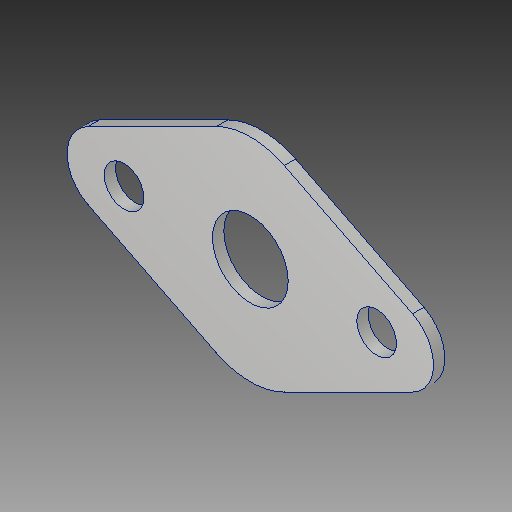
# Autodesk Inventor part: Maintient roulement
Saved by Autodesk Inventor 2017 (Build 210142000, 142)
## iProperties
Company: FABLAB Frenchmakers
Part Number: Maintient roulement
Material: Aluminium
Document SubType Name: Modeling
Designer: FABLAB Frenchmakers
Density: 2.7 g/cm^3
Appearance: Aluminium - Plat(2)
Mass: 0.653954 g
Surface Area: 6.35876 cm^2
Volume: 0.242205 cm^3
Stock Number: 1420-01-08
Project: 1420 Vauban 3D XL
Catalog Web Link: http://frenchmakers.com/
Autodesk Inventor part; units mm, degrees
ref_plane "YZ Plane" through (0, 0, 0) normal (1, 0, 0) x (0, 1, 0)
ref_plane "XZ Plane" through (0, 0, 0) normal (0, 1, 0) x (-1, 0, 0)
ref_plane "XY Plane" through (0, 0, 0) normal (0, 0, 1) x (1, 0, 0)
sketch "Esquisse1" plane through (0, 0, 0) normal (0, 0, 1) x (1, 0, 0)
  line L0 (-12.8425, 2.6828) -> (-2.685, 7.7657)
  line L1 (2.685, 7.7657) -> (12.8425, 2.6828)
  line L2 (12.8425, -2.6828) -> (2.685, -7.7657)
  line L3 (-2.685, -7.7657) -> (-12.8425, -2.6828)
  arc A0 (2.685, 7.7657) -> (-2.685, 7.7657) centre (0, 2.4) ccw
  arc A1 (-2.685, -7.7657) -> (2.685, -7.7657) centre (0, -2.4) ccw
  arc A2 (-12.8425, 2.6828) -> (-12.8425, -2.6828) centre (-11.5, 0) ccw
  arc A3 (12.8425, -2.6828) -> (12.8425, 2.6828) centre (11.5, 0) ccw
  point P0 (0, 0)
  point P1 (0, 9.1093)
  point P2 (18.2039, 0)
  point P3 (0, -9.1093)
  point P4 (-18.2039, 0)
  dimension "d0" = 6
  dimension "d1" = 3
  dimension "d2" = 29
  dimension "d3" = 16.8
  constraints: 8 end point, 8 point on circle, 8 point on line, 8 tangent, 4 centre point, 3 horizontal alignment, 2 equal length, 2 equal radius, 2 vertical alignment
  measures "d0" radius of A0
  measures "d1" radius of A2
extrude "Extrusion1" add sketch "Esquisse1" along normal blind 0.9
sketch "Esquisse2" plane through (0, 0, 0.9) normal (0, 0, 1) x (1, 0, 0)
  point P0 (0, 0)
  point P1 (0, 0)
  constraints: 1 coincident
hole "Perçage D6" at (0, 0, 0.9) direction (0, 0, -1) diameter 6 end through all
sketch "Esquisse3" plane through (0, 0, 0.9) normal (0, 0, 1) x (1, 0, 0)
  point P0 (0, 0)
  point P1 (-10, 0)
  point P2 (10, 0)
  dimension "d13" = 20
  dimension "d21" = 10
  constraints: 2 horizontal alignment
  measures "d13" distance of point (10, 0) point (-10, 0)
  measures "d21" distance of point (0, 0) point (10, 0)
hole "Perçage D3.15" at (-10, 0, 0.9) at (10, 0, 0.9) direction (0, 0, -1) diameter 3.15 end through all
equation "\"d21\" = 0.5 * d13"
